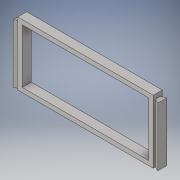
# Autodesk Inventor part: doveTailBar
Saved by Autodesk Inventor 2016 (Build 200138000, 138)
## iProperties
Created: 2015-11-04
Part Number: doveTailBar
Material: Generic
Document SubType Name: Modeling
Designer: rossmosier
Density: 1 g/cm^3
Appearance: Default
Author: rossmosier
Autodesk Inventor part; units mm, degrees
ref_plane "YZ Plane" through (0, 0, 0) normal (1, 0, 0) x (0, 1, 0)
ref_plane "XZ Plane" through (0, 0, 0) normal (0, 1, 0) x (-1, 0, 0)
ref_plane "XY Plane" through (0, 0, 0) normal (0, 0, 1) x (1, 0, 0)
sketch "Sketch1" plane through (0, 0, 0) normal (0, 1, 0) x (-1, 0, 0)
  line L0 (0, 0) -> (-190.5, 0)
  line L1 (-190.5, 0) -> (-190.5, -12.7)
  line L2 (-190.5, -12.7) -> (0, -12.7)
  line L3 (0, -12.7) -> (0, 0)
  dimension "d0" = 190.5
  dimension "d1" = 12.7
  constraints: 8 end point, 2 parallel, 1 horizontal, 1 perpendicular
  measures "d0" distance of L2.end L1.end
  measures "d1" distance of L1.end L0.end
extrude "Extrusion1" add sketch "Sketch1" along normal blind 88.9
sketch "Sketch2" plane through (0, 0, 0) normal (0, 1, 0) x (-1, 0, 0)
  line L0 (0, -12.7) -> (0, 0) construction
  line L1 (0, -12.6308) -> (0, 0) construction
  line L2 (0, -6.3154) -> (6.35, -6.3154) construction
  line L3 (6.35, 0) -> (6.35, -12.6308)
  line L4 (0, -6.3154) -> (0, -3.1658)
  line L5 (0, -6.3154) -> (0, -9.465)
  line L6 (0, -9.465) -> (6.35, -12.6308)
  line L7 (0, -3.1658) -> (6.35, 0)
  line L8 (-190.5, -12.7) -> (0, -12.7) construction
  line L9 (-95.25, -12.7) -> (-95.25, 0) construction
  line L10 (-190.5, -12.7) -> (-190.5, 0) construction
  line L11 (-196.85, 0) -> (-196.85, -12.6308)
  line L12 (-190.5, -9.465) -> (-196.85, -12.6308)
  line L13 (-190.5, -3.1658) -> (-196.85, 0)
  line L14 (-190.5, -9.465) -> (-190.5, -3.1658)
  line L15 (0, -9.465) -> (0, -3.1658)
  line L16 (-190.5, -9.465) -> (-196.85, -12.6308)
  line L17 (-196.85, 0) -> (-190.5, -3.1658)
  dimension "d4" = 6.35
  dimension "d5" = 3.1496
  dimension "d6" = 3.1496
  dimension "d9" = 12.6308
  constraints: 32 end point, 5 symmetric about line, 3 collinear, 3 point on line, 3 vertical, 2 midpoint, 1 horizontal
  measures "d4" distance of L2.start L2.end
  measures "d5" distance of L2.start L4.end
  measures "d6" distance of L2.start L5.end
  measures "d9" distance of L3.start L3.end
extrude "Extrusion2" add sketch "Sketch2" along normal blind 82.55
sketch "Sketch3" plane through (0, 0, 0) normal (0, 0, 1) x (1, 0, 0)
  line L0 (0, 0) -> (190.5, 0) projected
  line L1 (190.5, 0) -> (190.5, 88.9) projected
  line L2 (0, 88.9) -> (190.5, 88.9) projected
  line L3 (0, 0) -> (0, 88.9) projected
  line L4 (184.15, 82.55) -> (184.15, 6.35)
  line L5 (184.15, 6.35) -> (6.35, 6.35)
  line L6 (31.75, 82.55) -> (31.75, 6.35)
  line L7 (6.35, 6.35) -> (6.35, 82.55)
  line L8 (6.35, 82.55) -> (184.15, 82.55)
  line L9 (38.1, 82.55) -> (38.1, 6.35)
  line L10 (63.5, 82.55) -> (63.5, 6.35)
  line L11 (69.85, 82.55) -> (69.85, 6.35)
  line L12 (95.25, 82.55) -> (95.25, 6.35)
  line L13 (101.6, 82.55) -> (101.6, 6.35)
  line L14 (127, 82.55) -> (127, 6.35)
  line L15 (133.35, 82.55) -> (133.35, 6.35)
  line L16 (158.75, 82.55) -> (158.75, 6.35)
  line L17 (165.1, 82.55) -> (165.1, 6.35)
  line L18 (6.35, 82.55) -> (184.15, 82.55)
  line L19 (184.15, 82.55) -> (184.15, 6.35)
  line L20 (184.15, 6.35) -> (6.35, 6.35)
  line L21 (6.35, 6.35) -> (6.35, 82.55)
  dimension "d12" = 6.35
  dimension "d13" = 25.4
  dimension "d14" = 6.35
  dimension "d15" = 25.4
  dimension "d16" = 6.35
  dimension "d17" = 25.4
  dimension "d18" = 6.35
  dimension "d19" = 25.4
  dimension "d20" = 6.35
  constraints: 36 end point, 11 parallel, 2 perpendicular, 2 vertical, 1 horizontal, 1 point on line, 1 other
  measures "d12" distance between parallel lines of L6 L9
  measures "d13" distance between parallel lines of L9 L10
  measures "d14" distance between parallel lines of L10 L11
  measures "d15" distance between parallel lines of L11 L12
  measures "d16" distance between parallel lines of L12 L13
  measures "d17" distance between parallel lines of L13 L14
  measures "d18" distance between parallel lines of L14 L15
  measures "d19" distance between parallel lines of L15 L16
  measures "d20" distance between parallel lines of L16 L17
extrude "Extrusion3" cut sketch "Sketch3" against normal blind 76.2 contours L4 L5 L17 L8 | L17 L5 L16 L8 | L16 L5 L15 L8 | L15 L5 L14 L8 | L14 L5 L13 L8 | L13 L5 L12 L8 | L12 L5 L11 L8 | L11 L5 L10 L8 | L10 L5 L9 L8 | L9 L5 L6 L8 | L6 L5 L7 L8
body "Solid1"
